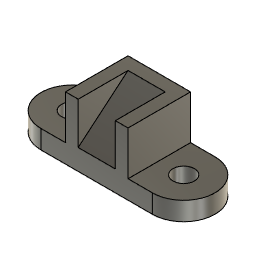
A2 (Autodesk Fusion 360 design; units mm, degrees)
Autodesk Fusion 360 part; units mm, degrees
sketch "Sketch1" plane through (0, 0, 0) normal (0, 0, 1) x (1, 0, 0)
  line L0 (57, -32) -> (-57, -32)
  line L1 (-57, 32) -> (57, 32)
  circle A0 centre (-57, 0) radius 11
  circle A1 centre (57, 0) radius 11
  arc A2 (-57, 32) -> (-57, -32) centre (-57, 0) ccw
  arc A3 (57, -32) -> (57, 32) centre (57, 0) ccw
  dimension "d1" = 114
  dimension "d2" = 64
  dimension "d5" = 64
  constraint horizontal L0
  constraint parallel L0 L1
  measures "d1" distance of L1.start L1.end
  measures "d2" distance of L0.end L1.start
  measures "d5" diameter of A3
extrude "Extrude1" add sketch "Sketch1" along normal blind 19
sketch "Sketch2" plane through (0, 0, 19) normal (0, 0, 1) x (-1, 0, 0)
  circle A0 centre (-57, 0) radius 11
  circle A1 centre (57, 0) radius 11
  arc A2 (57, -32) -> (57, 32) centre (57, 0) ccw
  line L0 (57, 32) -> (-57, 32)
  arc A3 (-57, 32) -> (-57, -32) centre (-57, 0) ccw
  line L1 (-57, -32) -> (57, -32)
  line L2 (109.1648, -142.7136) -> (36.9817, -142.7136)
  line L3 (36.9817, -142.7136) -> (36.9817, -79.8914)
  line L4 (36.9817, -79.8914) -> (109.1648, -79.8914)
  line L5 (109.1648, -79.8914) -> (109.1648, -142.7136)
  constraint horizontal L2
  constraint vertical L3
  constraint horizontal L4
  constraint vertical L5
sketch "Sketch3" plane through (0, 79.8914, 0) normal (0, -1, 0) x (1, 0, 0)
  line L0 (-109.1648, 19) -> (-36.9817, 19)
  line L1 (-36.9817, 19) -> (-36.9817, 119)
  line L2 (-36.9817, 119) -> (-109.1648, 119)
  line L3 (-109.1648, 119) -> (-109.1648, 19)
  line L4 (-91.5428, 119) -> (-50.2246, 119)
  line L5 (-50.2246, 119) -> (-50.2246, 19)
  line L6 (-50.2246, 19) -> (-91.5428, 19)
  line L7 (-91.5428, 19) -> (-91.5428, 119)
  constraint horizontal L4
  constraint vertical L5
  constraint horizontal L6
  constraint vertical L7
  constraint coincident L0 L5.end
  constraint coincident L2 L4.start
sketch "Sketch4" plane through (0, 0, 19) normal (0, 0, 1) x (-1, 0, 0)
  circle A0 centre (-57, 0) radius 11
  circle A1 centre (57, 0) radius 11
  arc A2 (57, -32) -> (57, 32) centre (57, 0) ccw
  line L0 (57, 32) -> (-57, 32)
  arc A3 (-57, 32) -> (-57, -32) centre (-57, 0) ccw
  line L1 (-57, -32) -> (57, -32)
  line L2 (32, 32) -> (-32, 32)
  line L3 (-32, 32) -> (-32, -32)
  line L4 (-32, -32) -> (32, -32)
  line L5 (32, -32) -> (32, 32)
  line L6 (32, 32) -> (-32, -32) construction
  line L7 (-32, 32) -> (32, -32) construction
  dimension "d18" = 64
  dimension "d19" = 64
  constraint horizontal L2
  constraint perpendicular L2 L3
  constraint parallel L2 L4
  constraint parallel L3 L5
  constraint coincident L6 origin
  constraint coincident L7 origin
  measures "d18" distance of L3.end L4.end
  measures "d19" distance of L2.end L3.end
extrude "Extrude4" add sketch "Sketch4" along normal blind 45 contours L0 L1 L2 L3 L4 L5
sketch "Sketch5" plane through (0, 0, 0) normal (0, 0, 1) x (1, 0, 0)
  line L0 (-215, 185) -> (-130, 185)
  line L1 (-130, 185) -> (-130, 110)
  line L2 (-130, 110) -> (-215, 110)
  line L3 (-215, 110) -> (-215, 185)
  constraint horizontal L0
  constraint vertical L1
  constraint horizontal L2
  constraint vertical L3
sketch "Sketch6" plane through (0, 0, 64) normal (0, 0, 1) x (-1, 0, 0)
  line L0 (32, -32) -> (32, 32)
  line L1 (32, 32) -> (-32, 32)
  line L2 (-32, 32) -> (-32, -32)
  line L3 (-32, -32) -> (32, -32)
  line L4 (19, 32) -> (-19, 32)
  line L5 (-19, 32) -> (-19, -19)
  line L6 (-19, -19) -> (19, -19)
  line L7 (19, -19) -> (19, 32)
  dimension "d24" = 38
  dimension "d25" = 51
  dimension "d26" = 13
  constraint horizontal L4
  constraint vertical L5
  constraint horizontal L6
  constraint vertical L7
  constraint coincident L1 L4.start
  measures "d24" distance of L4.start L4.end
  measures "d25" distance of L4.start L6.end
  measures "d26" distance of L0 L7
extrude "Extrude6" cut sketch "Sketch6" against normal blind 45 contours L1 L4 L5 L6 L7
draft "Draft2" angle 50 neutral plane through (0, 0, 64) pull (0, 0, 1) 1 faces at (6.3333, 19, 49)
equation "d20 = 64 mm - 19 mm"
